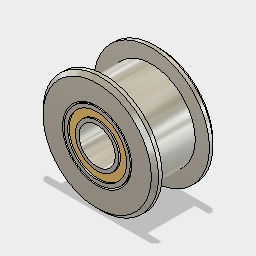
GT2 idler pulley (5 mm bore) v1 (Autodesk Fusion 360 design; units mm, degrees)
Autodesk Fusion 360 part; units mm, degrees
sketch "Sketch1" plane through (0, 0, 0) normal (0, 0, 1) x (1, 0, 0)
  circle A0 centre (0, 0) radius 6
  circle A1 centre (0, 0) radius 2.5
  dimension "d1" = 12
  dimension "d2" = 5
  measures "d1" diameter of A0
  measures "d2" diameter of A1
extrude "Extrude1" add sketch "Sketch1" along normal blind 6.5 makes body 1
sketch "Sketch2" plane through (0, 0, 6.5) normal (0, 0, 1) x (1, 0, 0)
  circle A0 centre (0, 0) radius 2.5
  circle A1 centre (0, 0) radius 6
  circle A2 centre (0, 0) radius 7.95
  dimension "d5" = 15.9
  measures "d5" diameter of A2
extrude "Extrude2" add sketch "Sketch2" along normal blind 1 contours A1 | A2 bodies 1
sketch "Sketch3" plane through (0, 0, 7.5) normal (0, 0, 1) x (1, 0, 0)
  circle A0 centre (0, 0) radius 2.5
  circle A1 centre (0, 0) radius 7.95
  circle A2 centre (0, 0) radius 4.75
  circle A3 centre (0, 0) radius 4.55
  circle A4 centre (0, 0) radius 4.05
  circle A5 centre (0, 0) radius 3
  dimension "d8" = 3.2
  dimension "d9" = 0.2
  dimension "d10" = 0.5
  dimension "d11" = 0.5
  measures "d8" distance of A1 A2
  measures "d9" distance of A2 A3
  measures "d10" distance of A3 A4
  measures "d11" distance of A0 A5
extrude "Extrude3" cut sketch "Sketch3" against normal blind 0.2 contours A2 bodies 1
chamfer "Chamfer1" distance 0.2 angle 45 1 edges at (-4.4286, 1.7177, 7.3) on bodies 1
extrude "Extrude4" cut sketch "Sketch3" against normal blind 0.2 contours A4 bodies 1
split "Split1" by plane through (0, 0, 6.5) normal (0, 0, -1) bodies 1 makes body 2 at (5.9925, -0.2991, 2.1667)
ref_plane "WorkPlane1" through (0, 0, 3.25) normal (0, 0, -1) x (-1, 0, 0)
mirror "Mirror1" about plane through (0, 0, 3.25) normal (0, 0, -1) of bodies 1 makes body 3
combine "Combine1" operation add target body 1 tool bodies 2 3
chamfer "Chamfer2" distance 0.5 angle 45 2 edges at (-7.412, -2.8748, 7.5) (-7.412, -2.8748, -1) on bodies 1
equation "d17 = ( -6.5 / 2 ) * 1 mm"
